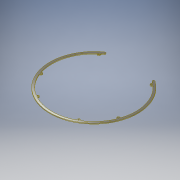
# Autodesk Inventor part: alu_ring_pesus
Saved by Autodesk Inventor 2018 (Build 220112000, 112)
## iProperties
Created: 2019-03-04
Part Number: alu_ring_pesus
Material: Aluminum 6061-AHC
Document SubType Name: Modeling
Designer: RedBots
Density: 2.7 g/cm^3
Appearance: Silber
Mass: 15.0871 g
Surface Area: 79.1705 cm^2
Volume: 5.58781 cm^3
Author: RedBots
Autodesk Inventor part; units mm, degrees
ref_plane "YZ Plane" through (0, 0, 0) normal (1, 0, 0) x (0, 1, 0)
ref_plane "XZ Plane" through (0, 0, 0) normal (0, 1, 0) x (-1, 0, 0)
ref_plane "XY Plane" through (0, 0, 0) normal (0, 0, 1) x (1, 0, 0)
sketch "Skizze1" plane through (0, 0, 0) normal (0, 0, 1) x (1, 0, 0)
  circle A0 centre (0, 0) radius 102 construction
  circle A1 centre (0, 0) radius 107 construction
  line L0 (0, 0) -> (107, 0) construction
  line L1 (0, 0) -> (107, 0) construction
  line L2 (0, 0) -> (107, 0) construction
  line L3 (0, 0) -> (107, 0) construction
  circle A2 centre (64.2788, 76.6044) radius 1.5
  circle A3 centre (93.9693, -34.202) radius 1.5
  circle A4 centre (50, -86.6025) radius 1.5
  line L4 (0, 0) -> (100, 0) construction
  line L5 (0, 0) -> (64.2788, 76.6044) construction
  line L6 (0, 0) -> (100, 0) construction
  line L7 (0, 0) -> (93.9693, -34.202) construction
  line L8 (0, 0) -> (100, 0) construction
  line L9 (0, 0) -> (50, -86.6025) construction
  line L10 (0, 0) -> (100, 0) construction
  arc A5 (61.9806, 78.5328) -> (66.5769, 74.6761) centre (64.2788, 76.6044) ccw
  line L11 (64.2788, 76.6044) -> (61.9806, 78.5328) construction
  line L12 (61.9806, 78.5328) -> (63.2378, 80.0311)
  line L13 (66.5769, 74.6761) -> (67.8341, 76.1744)
  arc A6 (94.9953, -31.3829) -> (92.9432, -37.0211) centre (93.9693, -34.202) ccw
  line L14 (93.9693, -34.202) -> (94.9953, -31.3829) construction
  line L15 (94.9953, -31.3829) -> (96.8332, -32.0519)
  line L16 (92.9432, -37.0211) -> (94.7811, -37.69)
  arc A7 (52.5981, -85.1025) -> (47.4019, -88.1025) centre (50, -86.6025) ccw
  line L17 (50, -86.6025) -> (52.5981, -85.1025) construction
  line L18 (52.5981, -85.1025) -> (53.576, -86.7964)
  line L19 (47.4019, -88.1025) -> (48.3799, -89.7964)
  line L20 (0, 0) -> (0, -102) construction
  circle A8 centre (-64.2788, 76.6044) radius 1.5
  circle A9 centre (-93.9693, -34.202) radius 1.5
  circle A10 centre (-50, -86.6025) radius 1.5
  arc A11 (-66.5769, 74.6761) -> (-61.9806, 78.5328) centre (-64.2788, 76.6044) ccw
  line L21 (-61.9806, 78.5328) -> (-63.2378, 80.0311)
  line L22 (-66.5769, 74.6761) -> (-67.8341, 76.1744)
  arc A12 (-92.9432, -37.0211) -> (-94.9953, -31.3829) centre (-93.9693, -34.202) ccw
  line L23 (-94.9953, -31.3829) -> (-96.8332, -32.0519)
  line L24 (-92.9432, -37.0211) -> (-94.7811, -37.69)
  arc A13 (-47.4019, -88.1025) -> (-52.5981, -85.1025) centre (-50, -86.6025) ccw
  line L25 (-52.5981, -85.1025) -> (-53.576, -86.7964)
  line L26 (-47.4019, -88.1025) -> (-48.3799, -89.7964)
  line L27 (0, 0) -> (-61, 87.909) construction
  line L28 (0, 0) -> (61, 87.909) construction
  line L29 (-61, 87.909) -> (61, 87.909) construction
  arc A14 (-58.1495, 83.8011) -> (-61, 87.909) centre (-59.5748, 85.8551) ccw
  arc A15 (61, 87.909) -> (58.1495, 83.8011) centre (59.5748, 85.8551) ccw
  arc A16 (-61, 87.909) -> (61, 87.909) centre (0, 0) ccw
  arc A17 (-58.1495, 83.8011) -> (-63.2378, 80.0311) centre (0, 0) ccw
  arc A18 (-67.8341, 76.1744) -> (-96.8332, -32.0519) centre (0, 0) ccw
  arc A19 (-94.7811, -37.69) -> (-53.576, -86.7964) centre (0, 0) ccw
  arc A20 (-48.3799, -89.7964) -> (48.3799, -89.7964) centre (0, 0) ccw
  arc A21 (53.576, -86.7964) -> (94.7811, -37.69) centre (0, 0) ccw
  arc A22 (96.8332, -32.0519) -> (67.8341, 76.1744) centre (0, 0) ccw
  arc A23 (63.2378, 80.0311) -> (58.1495, 83.8011) centre (0, 0) ccw
  dimension "d0" = 204
  dimension "d1" = 214
  dimension "d11" = 50
  dimension "d12" = 20
  dimension "d13" = 60
  dimension "d14" = 100
  dimension "d15" = 3
  dimension "d16" = 6
  dimension "d18" = 122
  dimension "d19" = 2.5
  constraints: 60 end point, 40 point on circle, 26 symmetric about line, 24 centre point, 15 coincident, 9 horizontal, 6 perpendicular, 5 equal length, 5 equal radius, 2 point on line, 1 vertical, 7 other
  measures "d0" diameter of A0
  measures "d1" diameter of A1
  measures "d11" angle of L6 L5
  measures "d12" angle of L7 L8
  measures "d13" angle of L9 L10
  measures "d14" distance of L0.start L5.end
  measures "d15" diameter of A2
  measures "d16" diameter of A5
  measures "d18" distance of L27.end L28.end
  measures "d19" radius of A14
extrude "Extrusion1" add sketch "Skizze1" along normal blind 2
fillet "Rundung1" radius 2 12 edges at (-63.2378, 80.0311, 1) (-94.7811, -37.69, 1) (-48.3799, -89.7964, 1) (53.576, -86.7964, 1) (96.8332, -32.0519, 1) (94.7811, -37.69, 1) (63.2378, 80.0311, 1) (67.8341, 76.1744, 1) (48.3799, -89.7964, 1) (-53.576, -86.7964, 1) (-96.8332, -32.0519, 1) (-67.8341, 76.1744, 1)
